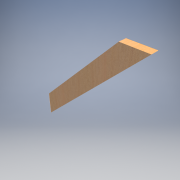
# Autodesk Inventor part: Back Angle Piece
Saved by Autodesk Inventor 2018 (Build 220112000, 112)
## iProperties
Created: 2016-08-30
Part Number: Back Angle Piece
Material: Wood
Document SubType Name: Modeling
Designer: jjsch
Density: 0.570257 g/cm^3
Appearance: Yellow Pine - Solid Natural Low Gloss
Mass: 1005.74 g
Surface Area: 1554.67 cm^2
Volume: 1763.66 cm^3
Author: jjsch
Autodesk Inventor part; units mm, degrees
ref_plane "YZ Plane" through (0, 0, 0) normal (1, 0, 0) x (0, 1, 0)
ref_plane "XZ Plane" through (0, 0, 0) normal (0, 1, 0) x (-1, 0, 0)
ref_plane "XY Plane" through (0, 0, 0) normal (0, 0, 1) x (1, 0, 0)
sketch "Sketch1" plane through (0, 0, 0) normal (0, 0, 1) x (1, 0, 0)
  line L0 (0, 0) -> (552.2858, 552.2858)
  line L1 (0, 0) -> (781.05, 0) construction
  line L2 (552.2858, 552.2858) -> (489.424, 615.1475)
  line L3 (489.424, 615.1475) -> (-62.8618, 62.8618)
  line L4 (-62.8618, 62.8618) -> (0, 0)
  line L5 (0, 125.7236) -> (0, 0)
  line L6 (552.2858, 552.2858) -> (426.5622, 552.2858)
  dimension "d8" = 781.05
  dimension "d9" = 45
  dimension "d10" = 88.9
  dimension "d11" = 90
  constraints: 14 end point, 3 perpendicular, 2 point on line, 1 equal length, 1 horizontal, 1 vertical
  measures "d8" distance of L0.start L0.end
  measures "d9" angle of L1 L0
  measures "d10" distance of L0.end L2.end
  measures "d11" angle of L3 L2
extrude "Extrusion1" add sketch "Sketch1" along normal blind 38.1 contours L5 L3 L6 L0
body "Solid1"
